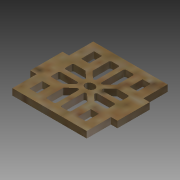
# Autodesk Inventor part: escbase
Saved by Autodesk Inventor 2012 (Build 160160000, 160)
## iProperties
Created: 2014-07-18
Part Number: escbase
Material: Default
Document SubType Name: Modeling
Designer: Anon
Density: 1 g/cm^3
Author: Anon
Autodesk Inventor part; units mm, degrees
ref_plane "YZ Plane" through (0, 0, 0) normal (1, 0, 0) x (0, 1, 0)
ref_plane "XZ Plane" through (0, 0, 0) normal (0, 1, 0) x (-1, 0, 0)
ref_plane "XY Plane" through (0, 0, 0) normal (0, 0, 1) x (1, 0, 0)
sketch "Sketch1" plane through (0, 0, 0) normal (0, 0, 1) x (1, 0, 0)
  line L0 (-23, 25) -> (23, 25)
  line L1 (23, 25) -> (23, 10)
  line L2 (23, 10) -> (27, 10)
  line L3 (27, 10) -> (27, -10)
  line L4 (27, -10) -> (23, -10)
  line L5 (23, -10) -> (23, -25)
  line L6 (23, -25) -> (-23, -25)
  line L7 (-23, -25) -> (-23, -10)
  line L8 (-23, -10) -> (-27, -10)
  line L9 (-27, -10) -> (-27, 10)
  line L10 (-27, 10) -> (-23, 10)
  line L11 (-23, 10) -> (-23, 25)
  point P0 (0, 0)
  dimension "d0" = 46
  dimension "d1" = 15
  dimension "d2" = 4
  dimension "d3" = 20
  dimension "d4" = 4
  dimension "d5" = 15
  dimension "d6" = 46
  dimension "d7" = 15
  dimension "d8" = 4
  dimension "d9" = 20
  dimension "d10" = 4
  dimension "d11" = 25
  dimension "d12" = 27
  constraints: 24 end point, 7 perpendicular, 3 parallel, 1 horizontal
  measures "d0" distance of L0.start L0.end
  measures "d1" distance of L0.end L1.end
  measures "d2" distance of L1.end L2.end
  measures "d3" distance of L2.end L3.end
  measures "d4" distance of L3.end L4.end
  measures "d5" distance of L4.end L5.end
  measures "d6" distance of L5.end L6.end
  measures "d7" distance of L6.end L7.end
  measures "d8" distance of L7.end L8.end
  measures "d9" distance of L8.end L9.end
  measures "d10" distance of L9.end L10.end
  measures "d11" distance from line of point (0, 0) L0
  measures "d12" distance from line of point (0, 0) L9
extrude "Base" add sketch "Sketch1" along normal blind 4
sketch "Sketch2" plane through (0, 0, 4) normal (0, 0, 1) x (1, 0, 0)
  line L0 (-17.5, 20) -> (-12.5, 20)
  line L1 (-12.5, 20) -> (-12.5, 12)
  line L2 (-12.5, 12) -> (-17.5, 12)
  line L3 (-17.5, 12) -> (-17.5, 20)
  point P0 (0, 0)
  dimension "d15" = 5
  dimension "d16" = 8
  dimension "d17" = 12.5
  dimension "d18" = 12
  constraints: 8 end point, 2 parallel, 1 horizontal, 1 perpendicular
  measures "d15" distance of L1.end L2.end
  measures "d16" distance between parallel lines of L0 L2
  measures "d17" distance from line of point (0, 0) L1
  measures "d18" distance from line of point (0, 0) L2
extrude "FrictionLocks" cut sketch "Sketch2" against normal blind 4
mirror "LockDoubler" about plane through (0, 0, 0) normal (0, 1, 0) of "FrictionLocks"
mirror "LockQuadrupler" about plane through (0, 0, 0) normal (1, 0, 0) of "FrictionLocks", "LockDoubler"
sketch "Sketch5" plane through (0, 0, 4) normal (0, 0, 1) x (1, 0, 0)
  line L0 (-17.5, 20) -> (-12.5, 20) projected
  line L1 (-12.5, 20) -> (-12.5, 12) projected
  line L2 (-12.5, 12) -> (-17.5, 12) projected
  line L3 (23, 10) -> (27, 10) projected
  line L4 (-7.5, 20) -> (-1.5, 20)
  line L5 (-1.5, 20) -> (-1.5, 1.5)
  line L6 (-1.5, 1.5) -> (-17.5, 1.5)
  line L7 (-17.5, 1.5) -> (-17.5, 7)
  line L8 (-17.5, 7) -> (-7.5, 7)
  line L9 (-7.5, 7) -> (-7.5, 20)
  point P0 (0, 0)
  dimension "d50" = 1.5
  dimension "d51" = 1.5
  dimension "d52" = 0
  dimension "d53" = 5
  dimension "d54" = 5
  dimension "d55" = 5
  constraints: 12 end point, 5 parallel, 1 perpendicular
  measures "d50" distance from line of point (0, 0) L6
  measures "d51" distance from line of point (0, 0) L5
  measures "d52" distance between parallel lines of L0 L4
  measures "d53" distance between parallel lines of L1 L9
  measures "d54" distance between parallel lines of L8 L2
  measures "d55" distance between parallel lines of L1 L7
extrude "WeightRelieve" cut sketch "Sketch5" against normal blind 4
sketch "Sketch6" plane through (0, 0, 4) normal (0, 0, 1) x (1, 0, 0)
  line L0 (-7.5, 7) -> (-7.5, 20) projected
  line L1 (-1.5, 20) -> (-1.5, 1.5) projected
  line L2 (-1.5, 1.5) -> (-17.5, 1.5) projected
  line L3 (-17.5, 7) -> (-7.5, 7) projected
  line L4 (0, 0) -> (-7.5, 7) construction
  line L5 (-7.9828, 9.5024) -> (0.1392, 1.9219) construction
  line L6 (-10.4569, 7.708) -> (-1.9362, -0.2447) construction
  line L7 (-7.5, 9.0518) -> (-1.5, 3.4518) construction
  line L8 (-1.5, 3.4518) -> (-7.5, 9.0518)
  line L9 (-7.5, 9.0518) -> (-7.5, 7)
  line L10 (-7.5, 7) -> (-9.6984, 7)
  line L11 (-9.6984, 7) -> (-3.8055, 1.5)
  line L12 (-3.8055, 1.5) -> (-1.5, 1.5)
  line L13 (-1.5, 1.5) -> (-1.5, 3.4518)
  dimension "d58" = 1.5
  dimension "d59" = 1.5
  constraints: 20 end point, 8 point on line, 3 collinear, 2 parallel, 1 perpendicular
  measures "d58" distance between parallel lines of L5 L4
  measures "d59" distance between parallel lines of L6 L4
extrude "SupportBeam" add sketch "Sketch6" against normal blind 4
fillet "SupportFillet" radius 1 8 edges at (-1.5, 3.4518, 2) (-1.5, 20, 2) (-9.6984, 7, 2) (-7.5, 9.0518, 2) (-7.5, 20, 2) (-3.8055, 1.5, 2) (-17.5, 7, 2) (-17.5, 1.5, 2)
mirror "RelieveDoubler" about plane through (0, 0, 0) normal (0, 1, 0) of "WeightRelieve", "SupportBeam", "SupportFillet"
mirror "RelieveQuadrupler" about plane through (0, 0, 0) normal (1, 0, 0) of "WeightRelieve", "SupportBeam", "SupportFillet", "RelieveDoubler"
sketch "Sketch7" plane through (0, 0, 4) normal (0, 0, 1) x (1, 0, 0)
  line L0 (6.3426, -1.5) -> (16.5, -1.5) projected
  ellipse E0 centre (0, 0) end of major axis (3, 0) minor radius 2.5
  dimension "d63" = 3
  dimension "d64" = 2.5
  constraints: 1 coincident, 1 horizontal, 2 other
extrude "CenterEllipse" cut sketch "Sketch7" against normal blind 4
equation "\"BendRadius\" = Thickness"
equation "\"BendReliefWidth\" = Thickness"
equation "\"BendReliefDepth\" = 0.5 * Thickness"
equation "\"CornerReliefSize\" = 4 * Thickness"
equation "\"MinimumRemnant\" = 2 * Thickness"
equation "\"TransitionRadius\" = BendRadius"
equation "\"JacobiRadiusSize\" = Thickness"
equation "\"GapSize\" = Thickness"
equation "\"Thickness\" = 0.5"
body "Solid1"
